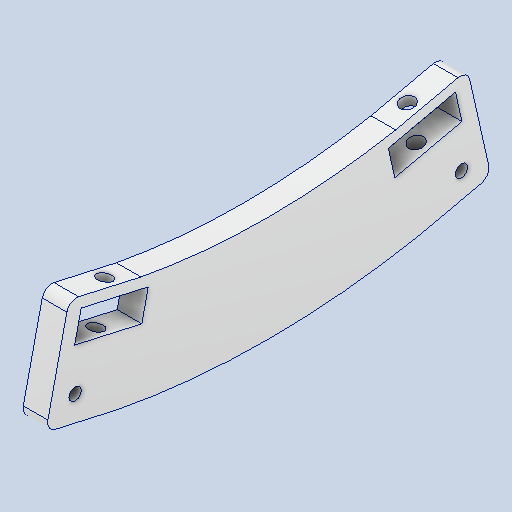
# Autodesk Inventor part: belt_liner_v2_Plate_14
Saved by Autodesk Inventor 2025.2 (Build 292293000, 293)
## iProperties
Created: 2025-01-06
Part Number: belt_liner_v2_Plate_14
Material: アルミニウム 6061
Document SubType Name: Modeling
Designer: haruy
Density: 2.7 g/cm^3
Appearance: アルミニウム - フラット
Mass: 22.219 g
Surface Area: 51.7738 cm^2
Volume: 8.22926 cm^3
Author: haruy
Autodesk Inventor part; units mm, degrees
ref_plane "YZ Plane" through (0, 0, 0) normal (1, 0, 0) x (0, 1, 0)
ref_plane "XZ Plane" through (0, 0, 0) normal (0, 1, 0) x (-1, 0, 0)
ref_plane "XY Plane" through (0, 0, 0) normal (0, 0, 1) x (1, 0, 0)
derived "base_weel-v2-Sketch-Base.ipt"
sketch "スケッチ1" plane through (0, 0, 0) normal (1, 0, 0) x (0, 1, 0)
  line L0 (-315, 315) -> (315, 315)
  line L1 (315, 315) -> (315, -315)
  line L2 (315, -315) -> (-315, -315)
  line L3 (-315, -315) -> (-315, 315)
  line L4 (-315, 315) -> (315, -315) construction
  line L5 (315, 315) -> (-315, -315) construction
  line L6 (-295, 218) -> (-295, -202)
  line L7 (-295, -202) -> (-315, -202)
  line L8 (-315, -202) -> (-315, 210)
  line L9 (242, 315) -> (-242, 315)
  line L10 (-242, 315) -> (-242, 295)
  line L11 (-242, 295) -> (242, 295)
  line L12 (242, 295) -> (242, 315)
  line L13 (-295, 218) -> (-295, 315)
  line L14 (0, 0) -> (-956.5973, 0)
  circle A0 centre (0, 0) radius 400
  line L15 (-330, 25) -> (-380, 25)
  line L16 (-380, 25) -> (-380, -25)
  line L17 (-380, -25) -> (-330, -25)
  line L18 (-330, -25) -> (-330, 25)
  line L19 (0, 0) -> (0, -630.9179)
  line L20 (-315, 40) -> (-395, 40)
  line L21 (-395, 40) -> (-395, 30)
  line L22 (-395, 30) -> (-315, 30)
  line L23 (-315, 30) -> (-315, 40)
  line L24 (-395, 30) -> (-385, 30)
  line L25 (-385, 30) -> (-385, 0)
  line L26 (-385, 0) -> (-395, 0)
  line L27 (-395, 0) -> (-395, 30)
  line L28 (295, 202) -> (315, 202)
  line L29 (315, 202) -> (315, -202)
  line L30 (315, -202) -> (295, -202)
  line L31 (295, -202) -> (295, 202)
  line L32 (-222.2183, -315) -> (242, -315)
  line L33 (242, -315) -> (242, -295)
  line L34 (242, -295) -> (-242, -295)
  line L35 (315, 315) -> (0, 0)
  line L36 (315, 125) -> (315, 145)
  circle A1 centre (512, 0) radius 122.5
  circle A2 centre (179.6905, 0) radius 600
  circle A3 centre (541.6815, 0) radius 200
  circle A4 centre (0, 0) radius 10
  arc A5 (0, 150) -> (0, -150) centre (0, 0) ccw
  arc A6 (0, 140) -> (0, -140) centre (0, 0) ccw
  line L37 (-146.3272, 32.9904) -> (-136.572, 30.791)
  line L38 (-137.5812, 37.6817) -> (-140.4404, 25)
  line L39 (-140.4404, 25) -> (-145.318, 26.0997)
  line L40 (-145.318, 26.0997) -> (-142.4588, 38.7814)
  line L41 (-142.4588, 38.7814) -> (-137.5812, 37.6817)
  arc A7 (-29.1302, 142.0438) -> (-29.1302, -142.0438) centre (0, 0) ccw
  circle A8 centre (-151.4904, 39.2799) radius 6.5 construction
  circle A9 centre (-129.0401, 34.2184) radius 6.5 construction
  circle A10 centre (-129.0401, 34.2184) radius 1.5 construction
  circle A11 centre (-151.4904, 39.2799) radius 1.5 construction
  line L42 (-30.1668, 22.5) -> (-174.1362, 22.5)
  line L43 (-174.1362, 22.5) -> (-174.1362, 7.5)
  line L44 (-174.1362, 7.5) -> (-30.1668, 7.5)
  line L45 (-30.1668, 7.5) -> (-30.1668, 22.5)
  circle A12 centre (-129.0401, -34.2184) radius 6.5 construction
  circle A13 centre (-129.0401, -34.2184) radius 1.5 construction
  line L46 (-142.4588, -38.7814) -> (-137.5812, -37.6817)
  line L47 (-145.318, -26.0997) -> (-142.4588, -38.7814)
  line L48 (-137.5812, -37.6817) -> (-140.4404, -25)
  line L49 (-140.4404, -25) -> (-145.318, -26.0997)
  circle A14 centre (-151.4904, -39.2799) radius 6.5 construction
  circle A15 centre (-151.4904, -39.2799) radius 1.5 construction
  line L50 (-146.3272, -32.9904) -> (-136.572, -30.791)
  line L51 (-30.1668, -22.5) -> (-174.1362, -22.5)
  line L52 (-174.1362, -7.5) -> (-30.1668, -7.5)
  line L53 (-30.1668, -7.5) -> (-30.1668, -22.5)
  line L54 (-174.1362, -22.5) -> (-174.1362, -7.5)
  line L55 (-151.4904, 39.2799) -> (-129.0401, 34.2184) construction
  line L56 (-129.0401, 34.2184) -> (-129.59, 31.7796) construction
  line L57 (-129.59, 31.7796) -> (-152.0402, 36.8412) construction
  line L58 (-152.0402, 36.8412) -> (-151.4904, 39.2799) construction
  line L59 (-129.0401, 34.2184) -> (-151.4904, 39.2799) construction
  line L60 (-151.4904, 39.2799) -> (-150.9405, 41.7187) construction
  line L61 (-150.9405, 41.7187) -> (-128.4903, 36.6572) construction
  line L62 (-128.4903, 36.6572) -> (-129.0401, 34.2184) construction
  line L63 (-128.4903, 36.6572) -> (-129.59, 31.7796) construction
  line L64 (-129.59, 31.7796) -> (-117.8838, 29.1404) construction
  line L65 (-117.8838, 29.1404) -> (-116.7841, 34.0179) construction
  line L66 (-116.7841, 34.0179) -> (-128.4903, 36.6572) construction
  line L67 (-150.9405, 41.7187) -> (-152.0402, 36.8412) construction
  line L68 (-152.0402, 36.8412) -> (-163.7464, 39.4804) construction
  line L69 (-163.7464, 39.4804) -> (-162.6467, 44.358) construction
  line L70 (-162.6467, 44.358) -> (-150.9405, 41.7187) construction
  line L71 (-155.2683, 45.2572) -> (-128.9412, 39.3216)
  line L72 (-128.9412, 39.3216) -> (-132.2403, 24.6889)
  line L73 (-132.2403, 24.6889) -> (-158.5673, 30.6245)
  line L74 (-158.5673, 30.6245) -> (-155.2683, 45.2572)
  line L75 (-128.9412, -39.3216) -> (-132.2403, -24.6889)
  line L76 (-155.2683, -45.2572) -> (-128.9412, -39.3216)
  line L77 (-132.2403, -24.6889) -> (-158.5673, -30.6245)
  line L78 (-158.5673, -30.6245) -> (-155.2683, -45.2572)
  arc A16 (-132.2403, 24.6889) -> (-132.2403, -24.6889) centre (0, 0) ccw
  arc A17 (-158.5673, 30.6245) -> (-158.5673, -30.6245) centre (0, 0) ccw
  circle A18 centre (-152.5, 15) radius 1.25
  line L79 (-145, 0) -> (-145, 74.7382) construction
  circle A19 centre (-137.5, 15) radius 1.25
  circle A20 centre (-137.5, -15) radius 1.25
  circle A21 centre (-152.5, -15) radius 1.25
  circle A22 centre (-151.4904, 39.2799) radius 1.25
  circle A23 centre (-129.0401, 34.2184) radius 1.25
  line L80 (-136.9835, 38.0595) -> (-140.0626, 24.4023)
  line L81 (-140.0626, 24.4023) -> (-145.9157, 25.7219)
  line L82 (-145.9157, 25.7219) -> (-142.8366, 39.3791)
  line L83 (-142.8366, 39.3791) -> (-136.9835, 38.0595)
  circle A24 centre (-151.4904, -39.2799) radius 1.25
  circle A25 centre (-129.0401, -34.2184) radius 1.25
  line L84 (-136.9835, -38.0595) -> (-140.0626, -24.4023)
  line L85 (-140.0626, -24.4023) -> (-145.9157, -25.7219)
  line L86 (-145.9157, -25.7219) -> (-142.8366, -39.3791)
  line L87 (-142.8366, -39.3791) -> (-136.9835, -38.0595)
  line L88 (0, 0) -> (0, 140)
  line L89 (0, 0) -> (-47.8828, 131.557)
  line L90 (0, 140) -> (0, 150)
  line L91 (-137.5846, 25.8938) -> (-134.2855, 40.5265)
  line L92 (-137.5846, -25.8938) -> (-134.2855, -40.5265)
  circle A26 centre (0, 0) radius 20
  line L93 (295, 45) -> (-295, 45)
  line L94 (-295, 45) -> (-295, 25)
  line L95 (-295, 25) -> (295, 25)
  line L96 (295, 25) -> (295, 45)
  line L97 (-40, 295) -> (-50, 295)
  line L98 (-50, 295) -> (-50, 45)
  line L99 (-50, 45) -> (-40, 45)
  line L100 (-40, 45) -> (-40, 295)
  line L101 (-50, -295) -> (-50, -45)
  line L102 (-40, -45) -> (-40, -295)
  line L103 (295, -45) -> (-295, -45)
  line L104 (-295, -25) -> (295, -25)
  line L105 (-40, 45) -> (-40, -45)
  line L106 (40, 45) -> (40, -45)
  circle A27 centre (20, 35) radius 1.5
  circle A28 centre (-20, 35) radius 1.5
  circle A29 centre (-20, -35) radius 1.5
  circle A30 centre (20, -35) radius 1.5
  circle A31 centre (-45, 125) radius 1.5
  circle A32 centre (-45, 125) radius 5
  circle A33 centre (-130, 35) radius 5
  circle A34 centre (-130, 35) radius 1.5
  line L107 (-40, 134.1641) -> (-40, 125)
  line L108 (-50, 125) -> (-50, 130.767)
  line L109 (-137.7498, 25) -> (-127.5801, 30.6246)
  line L110 (-132.5707, 45) -> (-126.366, 38.4342)
  line L111 (-40, -134.1641) -> (-40, -125)
  circle A35 centre (-45, -125) radius 5
  circle A36 centre (-45, -125) radius 1.5
  line L112 (-50, -125) -> (-50, -130.767)
  line L113 (-132.5707, -45) -> (-126.366, -38.4342)
  circle A37 centre (-130, -35) radius 5
  circle A38 centre (-130, -35) radius 1.5
  line L114 (-137.7498, -25) -> (-127.5801, -30.6246)
  line L115 (-242, -295) -> (-242, -315)
  line L116 (242, 315) -> (222, 315)
  line L117 (222, 315) -> (222, 295)
  line L118 (222, 295) -> (242, 295)
  line L119 (242, 295) -> (242, 315)
  line L120 (242, -315) -> (222, -315)
  line L121 (222, -315) -> (222, -295)
  line L122 (222, -295) -> (242, -295)
  line L123 (242, -295) -> (242, -315)
  line L124 (197, 295) -> (295, 197)
  line L125 (295, 197) -> (284.3934, 186.3934)
  line L126 (284.3934, 186.3934) -> (186.3934, 284.3934)
  line L127 (186.3934, 284.3934) -> (197, 295)
  line L128 (197, 295) -> (197, 315)
  line L129 (197.9167, 294.0833) -> (187.3101, 283.4767)
  line L130 (198.2703, 272.5165) -> (272.5165, 198.2703)
  line L131 (272.5165, 198.2703) -> (231.5043, 157.2581)
  line L132 (231.5043, 157.2581) -> (157.2581, 231.5043)
  line L133 (157.2581, 231.5043) -> (198.2703, 272.5165)
  line L134 (290.9013, 201.0987) -> (280.2947, 190.4921)
  line L135 (93.7624, 295) -> (295, 93.7624)
  line L136 (295, 93.7624) -> (284.3934, 83.1558)
  line L137 (284.3934, 83.1558) -> (83.1558, 284.3934)
  line L138 (214.1802, 277.8198) -> (203.5736, 267.2132)
  line L139 (277.8198, 214.1802) -> (267.2132, 203.5736)
  circle A39 centre (199.6845, 281.7089) radius 1.5
  circle A40 centre (213.8266, 267.5668) radius 1.5
  line L140 (186.3934, 284.3934) -> (175.7868, 295)
  circle A41 centre (187, 305) radius 1.5
  circle A42 centre (177, 305) radius 1.5
  line L141 (172, 315) -> (172, 295)
  line L142 (93.7624, 295) -> (93.7624, 295)
  line L143 (93.7624, 295) -> (93.7624, 315)
  line L144 (83.1558, 284.3934) -> (72.5492, 295)
  line L145 (68.7624, 315) -> (68.7624, 295)
  line L146 (284.3934, 186.3934) -> (295, 175.7868)
  line L147 (295, 197) -> (315, 197)
  line L148 (295, 93.7624) -> (295, 93.7624)
  line L149 (284.3934, 83.1558) -> (295, 72.5492)
  line L150 (-197, 295) -> (-197, 315)
  line L151 (-172, 315) -> (-172, 295)
  line L152 (-93.7624, 295) -> (-93.7624, 315)
  line L153 (-68.7624, 315) -> (-68.7624, 295)
  line L154 (-83.1558, 284.3934) -> (-72.5492, 295)
  line L155 (-93.7624, 295) -> (-295, 93.7624)
  line L156 (-83.1558, 284.3934) -> (-93.7624, 295)
  line L157 (-284.3934, 83.1558) -> (-83.1558, 284.3934)
  line L158 (-295, 93.7624) -> (-284.3934, 83.1558)
  line L159 (-284.3934, 83.1558) -> (-295, 72.5492)
  line L160 (-272.5165, 198.2703) -> (-231.5043, 157.2581)
  line L161 (-157.2581, 231.5043) -> (-198.2703, 272.5165)
  line L162 (-284.3934, 186.3934) -> (-186.3934, 284.3934)
  line L163 (-186.3934, 284.3934) -> (-175.7868, 295)
  line L164 (-197, 295) -> (-295, 197)
  line L165 (-197.9167, 294.0833) -> (-187.3101, 283.4767)
  line L166 (-214.1802, 277.8198) -> (-203.5736, 267.2132)
  line L167 (-290.9013, 201.0987) -> (-280.2947, 190.4921)
  line L168 (-284.3934, 186.3934) -> (-295, 175.7868)
  line L169 (-295, 197) -> (-315, 197)
  line L170 (-93.7624, -295) -> (-295, -93.7624)
  line L171 (-284.3934, -83.1558) -> (-83.1558, -284.3934)
  line L172 (-295, -93.7624) -> (-284.3934, -83.1558)
  line L173 (-197, -295) -> (-295, -197)
  line L174 (-284.3934, -186.3934) -> (-186.3934, -284.3934)
  line L175 (-290.9013, -201.0987) -> (-280.2947, -190.4921)
  line L176 (-214.1802, -277.8198) -> (-203.5736, -267.2132)
  line L177 (-197.9167, -294.0833) -> (-187.3101, -283.4767)
  line L178 (-83.1558, -284.3934) -> (-93.7624, -295)
  line L179 (284.3934, -83.1558) -> (83.1558, -284.3934)
  line L180 (83.1558, -284.3934) -> (93.7624, -295)
  line L181 (93.7624, -295) -> (295, -93.7624)
  line L182 (284.3934, -186.3934) -> (186.3934, -284.3934)
  line L183 (197.9167, -294.0833) -> (187.3101, -283.4767)
  line L184 (197, -295) -> (295, -197)
  line L185 (290.9013, -201.0987) -> (280.2947, -190.4921)
  line L186 (295, -93.7624) -> (284.3934, -83.1558)
  line L187 (242, 295) -> (222, 295)
  arc A43 (0, 86) -> (0, -86) centre (0, 0) ccw
  circle A44 centre (-90.8667, 48.5) radius 21
  circle A45 centre (0, 0) radius 124
  circle A46 centre (-90.8667, 48.5) radius 17
  arc A47 (40.4951, 75.8693) -> (0, 86) centre (0, 0) ccw
  line L188 (-40, 45) -> (-50, 45)
  line L189 (-50, 45) -> (-50, -45)
  line L190 (-50, -45) -> (-40, -45)
  line L191 (-40, -45) -> (-40, 45)
  line L192 (-40, 295) -> (-50, 295)
  line L193 (-50, 295) -> (-50, 315)
  line L194 (-50, 315) -> (-40, 315)
  line L195 (-40, 315) -> (-40, 295)
  line L196 (-40, -295) -> (-50, -295)
  line L197 (-50, -295) -> (-50, -315)
  line L198 (-50, -315) -> (-40, -315)
  line L199 (-40, -315) -> (-40, -295)
  line L200 (40, -315) -> (40, -295)
  line L201 (50, -295) -> (50, -315)
  line L202 (50, -295) -> (50, -45)
  line L203 (40, -45) -> (40, -295)
  line L204 (40, -45) -> (40, 45)
  line L205 (50, 45) -> (50, -45)
  line L206 (40, 45) -> (40, 295)
  line L207 (50, 295) -> (50, 45)
  line L208 (40, 315) -> (40, 295)
  line L209 (50, 295) -> (50, 315)
  line L210 (-40.4092, 123.019) -> (-35, 135.5544)
  line L211 (-48.7417, 121.6834) -> (-55, 128.7439)
  line L212 (-40.4092, -123.019) -> (-35, -135.5544)
  line L213 (-48.7417, -121.6834) -> (-55, -128.7439)
  arc A48 (40.4951, 75.8693) -> (-40.4951, -75.8693) centre (0, 0) ccw
  circle A49 centre (0, 0) radius 86 construction
  circle A50 centre (0, 0) radius 78.5
  circle A51 centre (-45, 58) radius 1.5
  circle A52 centre (-45, 58) radius 5
  circle A53 centre (45, 58) radius 5
  circle A54 centre (45, 58) radius 1.5
  line L214 (46.5549, 53.2479) -> (55, 56.0112)
  line L215 (40.325, 56.2267) -> (35, 70.2656)
  line L216 (50, 60.5165) -> (50, 69.9714)
  arc A55 (50, 69.9714) -> (40.4951, 75.8693) centre (0, 0) ccw
  line L217 (-40.325, 56.2267) -> (-35, 70.2656)
  line L218 (-46.5549, 53.2479) -> (-55, 56.0112)
  line L219 (-40.325, -56.2267) -> (-35, -70.2656) construction
  circle A56 centre (-45, -58) radius 5
  line L220 (-46.5549, -53.2479) -> (-55, -56.0112)
  circle A57 centre (-45, -58) radius 1.5
  line L221 (-40, -67.5444) -> (-40, -76.1315)
  arc A58 (-40.526, -75.8528) -> (-40, -76.1315) centre (0, 0) ccw
  line L222 (-40, -76.1315) -> (-40, -58)
  line L223 (222.6655, 269.3345) -> (212.0589, 258.7279)
  line L224 (269.3345, 222.6655) -> (258.7279, 212.0589)
  circle A59 centre (267.5668, 213.8266) radius 1.5
  circle A60 centre (281.7089, 199.6845) radius 1.5
  line L225 (294.0833, 197.9167) -> (283.4767, 187.3101)
  line L226 (315, 172) -> (295, 172)
  circle A61 centre (305, 177) radius 1.5
  circle A62 centre (305, 187) radius 1.5
  line L227 (295, 197) -> (315, 197)
  circle A63 centre (83.7624, 305) radius 1.5
  circle A64 centre (73.7624, 305) radius 1.5
  line L228 (197.9167, 294.0833) -> (94.6791, 294.0833)
  line L229 (187.3101, 283.4767) -> (84.0725, 283.4767)
  line L230 (94.6791, 294.0833) -> (84.0725, 283.4767)
  circle A65 centre (96.4469, 281.7089) radius 1.5
  circle A66 centre (110.5891, 267.5668) radius 1.5
  line L231 (119.4279, 269.3345) -> (108.8213, 258.7279)
  line L232 (295, 93.7624) -> (315, 93.7624)
  line L233 (315, 68.7624) -> (295, 68.7624)
  circle A67 centre (305, 73.7624) radius 1.5
  circle A68 centre (305, 83.7624) radius 1.5
  line L234 (294.0833, 94.6791) -> (283.4767, 84.0725)
  circle A69 centre (281.7089, 96.4469) radius 1.5
  circle A70 centre (267.5668, 110.5891) radius 1.5
  line L235 (269.3345, 119.4279) -> (258.7279, 108.8213)
  line L236 (-197, 295) -> (-197, 315)
  line L237 (-172, 315) -> (-172, 295)
  circle A71 centre (-177, 305) radius 1.5
  circle A72 centre (-187, 305) radius 1.5
  line L238 (-197.9167, 294.0833) -> (-187.3101, 283.4767)
  circle A73 centre (-199.6845, 281.7089) radius 1.5
  line L239 (-214.1802, 277.8198) -> (-203.5736, 267.2132)
  circle A74 centre (-213.8266, 267.5668) radius 1.5
  line L240 (-222.6655, 269.3345) -> (-212.0589, 258.7279)
  circle A75 centre (-267.5668, 213.8266) radius 1.5
  line L241 (-269.3345, 222.6655) -> (-258.7279, 212.0589)
  circle A76 centre (-281.7089, 199.6845) radius 1.5
  line L242 (-294.0833, 197.9167) -> (-283.4767, 187.3101)
  line L243 (-295, 197) -> (-315, 197)
  circle A77 centre (-305, 187) radius 1.5
  circle A78 centre (-305, 177) radius 1.5
  line L244 (-315, 172) -> (-295, 172)
  line L245 (-295, 93.7624) -> (-315, 93.7624)
  line L246 (-315, 68.7624) -> (-295, 68.7624)
  circle A79 centre (-305, 73.7624) radius 1.5
  circle A80 centre (-305, 83.7624) radius 1.5
  line L247 (-294.0833, 94.6791) -> (-283.4767, 84.0725)
  circle A81 centre (-281.7089, 96.4469) radius 1.5
  circle A82 centre (-267.5668, 110.5891) radius 1.5
  line L248 (-269.3345, 119.4279) -> (-258.7279, 108.8213)
  line L249 (-119.4279, 269.3345) -> (-108.8213, 258.7279)
  circle A83 centre (-110.5891, 267.5668) radius 1.5
  circle A84 centre (-96.4469, 281.7089) radius 1.5
  line L250 (-94.6791, 294.0833) -> (-84.0725, 283.4767)
  line L251 (-93.7624, 295) -> (-93.7624, 315)
  line L252 (-68.7624, 315) -> (-68.7624, 295)
  circle A85 centre (-73.7624, 305) radius 1.5
  circle A86 centre (-83.7624, 305) radius 1.5
  line L253 (-295, -197) -> (-315, -197)
  circle A87 centre (-305, -187) radius 1.5
  circle A88 centre (-305, -177) radius 1.5
  line L254 (-315, -172) -> (-295, -172)
  line L255 (-294.0833, -197.9167) -> (-283.4767, -187.3101)
  circle A89 centre (-281.7089, -199.6845) radius 1.5
  circle A90 centre (-267.5668, -213.8266) radius 1.5
  line L256 (-269.3345, -222.6655) -> (-258.7279, -212.0589)
  line L257 (-222.6655, -269.3345) -> (-212.0589, -258.7279)
  circle A91 centre (-213.8266, -267.5668) radius 1.5
  circle A92 centre (-199.6845, -281.7089) radius 1.5
  line L258 (-197.9167, -294.0833) -> (-187.3101, -283.4767)
  line L259 (-197, -295) -> (-197, -315)
  circle A93 centre (-187, -305) radius 1.5
  circle A94 centre (-177, -305) radius 1.5
  line L260 (-172, -315) -> (-172, -295)
  line L261 (-295, -93.7624) -> (-315, -93.7624)
  circle A95 centre (-305, -83.7624) radius 1.5
  circle A96 centre (-305, -73.7624) radius 1.5
  line L262 (-315, -68.7624) -> (-295, -68.7624)
  line L263 (-294.0833, -94.6791) -> (-283.4767, -84.0725)
  circle A97 centre (-281.7089, -96.4469) radius 1.5
  circle A98 centre (-267.5668, -110.5891) radius 1.5
  line L264 (-269.3345, -119.4279) -> (-258.7279, -108.8213)
  line L265 (-119.4279, -269.3345) -> (-108.8213, -258.7279)
  circle A99 centre (-110.5891, -267.5668) radius 1.5
  circle A100 centre (-96.4469, -281.7089) radius 1.5
  line L266 (-94.6791, -294.0833) -> (-84.0725, -283.4767)
  line L267 (-93.7624, -295) -> (-93.7624, -315)
  circle A101 centre (-83.7624, -305) radius 1.5
  circle A102 centre (-73.7624, -305) radius 1.5
  line L268 (-68.7624, -315) -> (-68.7624, -295)
  line L269 (68.7624, -315) -> (68.7624, -295)
  circle A103 centre (73.7624, -305) radius 1.5
  circle A104 centre (83.7624, -305) radius 1.5
  line L270 (93.7624, -295) -> (93.7624, -315)
  line L271 (94.6791, -294.0833) -> (84.0725, -283.4767)
  circle A105 centre (96.4469, -281.7089) radius 1.5
  circle A106 centre (110.5891, -267.5668) radius 1.5
  line L272 (119.4279, -269.3345) -> (108.8213, -258.7279)
  line L273 (172, -315) -> (172, -295)
  circle A107 centre (177, -305) radius 1.5
  circle A108 centre (187, -305) radius 1.5
  line L274 (197, -295) -> (197, -315)
  line L275 (197.9167, -294.0833) -> (187.3101, -283.4767)
  circle A109 centre (199.6845, -281.7089) radius 1.5
  circle A110 centre (213.8266, -267.5668) radius 1.5
  line L276 (222.6655, -269.3345) -> (212.0589, -258.7279)
  line L277 (269.3345, -222.6655) -> (258.7279, -212.0589)
  circle A111 centre (267.5668, -213.8266) radius 1.5
  circle A112 centre (281.7089, -199.6845) radius 1.5
  line L278 (294.0833, -197.9167) -> (283.4767, -187.3101)
  line L279 (295, -197) -> (315, -197)
  circle A113 centre (305, -187) radius 1.5
  circle A114 centre (305, -177) radius 1.5
  line L280 (315, -172) -> (295, -172)
  line L281 (295, -93.7624) -> (315, -93.7624)
  circle A115 centre (305, -83.7624) radius 1.5
  circle A116 centre (305, -73.7624) radius 1.5
  line L282 (315, -68.7624) -> (295, -68.7624)
  line L283 (294.0833, -94.6791) -> (283.4767, -84.0725)
  circle A117 centre (281.7089, -96.4469) radius 1.5
  line L284 (269.3345, -119.4279) -> (258.7279, -108.8213)
  circle A118 centre (267.5668, -110.5891) radius 1.5
  line L285 (-295, 202) -> (-315, 202)
  line L286 (265, 45) -> (265, 25)
  circle A119 centre (275, 35) radius 1.5
  circle A120 centre (285, 35) radius 1.5
  circle A121 centre (305, 35) radius 1.5
  circle A122 centre (305, 25) radius 1.5
  line L287 (295, 25) -> (315, 25)
  line L288 (265, -45) -> (265, -25)
  circle A123 centre (275, -35) radius 1.5
  circle A124 centre (285, -35) radius 1.5
  circle A125 centre (305, -35) radius 1.5
  circle A126 centre (305, -25) radius 1.5
  circle A127 centre (-305, -25) radius 1.5
  circle A128 centre (-305, -35) radius 1.5
  circle A129 centre (-285, -35) radius 1.5
  circle A130 centre (-275, -35) radius 1.5
  line L289 (-265, -45) -> (-265, -25)
  line L290 (-265, 45) -> (-265, 25)
  circle A131 centre (-275, 35) radius 1.5
  circle A132 centre (-285, 35) radius 1.5
  circle A133 centre (-305, 35) radius 1.5
  circle A134 centre (-305, 25) radius 1.5
  circle A135 centre (48, 345) radius 44
  circle A136 centre (-50, 345) radius 44
  circle A137 centre (-50, 345) radius 15
  line L291 (295, 45) -> (315, 45)
  line L292 (295, 15) -> (315, 15)
  line L293 (-315, 45.5) -> (-390, 45.5)
  line L294 (-390, 45.5) -> (-390, 0)
  line L295 (-390, 0) -> (-315, 0)
  line L296 (-315, 0) -> (-315, 45.5)
  circle A138 centre (-305, 48) radius 1.5
  circle A139 centre (-305, -48) radius 1.5
  line L297 (114.7878, 210) -> (54.7878, 210)
  line L298 (54.7878, 210) -> (54.7878, 270)
  line L299 (54.7878, 270) -> (114.7878, 270)
  line L300 (114.7878, 270) -> (114.7878, 210)
  line L301 (34.7878, 210) -> (-25.2122, 210)
  line L302 (-25.2122, 210) -> (-25.2122, 270)
  line L303 (-25.2122, 270) -> (34.7878, 270)
  line L304 (34.7878, 270) -> (34.7878, 210)
  line L305 (-45.2122, 250) -> (-115.2122, 250)
  line L306 (-115.2122, 250) -> (-115.2122, 266)
  line L307 (-115.2122, 266) -> (-45.2122, 266)
  line L308 (-45.2122, 266) -> (-45.2122, 250)
  line L309 (-50.2122, 214) -> (-110.2122, 214)
  line L310 (-110.2122, 214) -> (-110.2122, 230)
  line L311 (-110.2122, 230) -> (-50.2122, 230)
  line L312 (-50.2122, 230) -> (-50.2122, 214)
  circle A140 centre (0, 0) radius 175.5
  line L313 (-185, -89) -> (-302, -89)
  line L314 (-302, -89) -> (-302, 89)
  line L315 (-302, 89) -> (-185, 89)
  line L316 (-185, 89) -> (-185, -89)
  line L317 (287, -17.7878) -> (205, -17.7878)
  line L318 (205, -17.7878) -> (205, 79.2122)
  line L319 (205, 79.2122) -> (287, 79.2122)
  line L320 (287, 79.2122) -> (287, -17.7878)
  line L321 (284.5, -114.7878) -> (207.5, -114.7878)
  line L322 (207.5, -114.7878) -> (207.5, -37.7878)
  line L323 (207.5, -37.7878) -> (284.5, -37.7878)
  line L324 (284.5, -37.7878) -> (284.5, -114.7878)
  line L325 (281, 99.2122) -> (211, 99.2122)
  line L326 (211, 99.2122) -> (211, 115.2122)
  line L327 (211, 115.2122) -> (281, 115.2122)
  line L328 (281, 115.2122) -> (281, 99.2122)
  line L329 (137.7122, 315) -> (-137.7122, 315)
  line L330 (-137.7122, 315) -> (-137.7122, 185)
  line L331 (-137.7122, 185) -> (137.7122, 185)
  line L332 (137.7122, 185) -> (137.7122, 315)
  line L333 (315, -137.7122) -> (185, -137.7122)
  line L334 (185, -137.7122) -> (185, 137.7122)
  line L335 (185, 137.7122) -> (315, 137.7122)
  line L336 (315, 137.7122) -> (315, -137.7122)
  line L337 (258.7782, 137.7122) -> (278.7782, 137.7122)
  line L338 (278.7782, 137.7122) -> (278.7782, 127.7122)
  line L339 (278.7782, 127.7122) -> (258.7782, 127.7122)
  line L340 (258.7782, 127.7122) -> (258.7782, 137.7122)
  circle A141 centre (268.7782, 132.7122) radius 1.5
  line L341 (278.7782, 137.7122) -> (231.1981, 137.7122)
  line L342 (231.1981, 137.7122) -> (231.1981, 147.7122)
  line L343 (231.1981, 147.7122) -> (278.7782, 147.7122)
  line L344 (278.7782, 147.7122) -> (278.7782, 137.7122)
  line L345 (255.1924, 112.3568) -> (233.9792, 133.57)
  line L346 (233.9792, 133.57) -> (230.4437, 130.0345)
  line L347 (230.4437, 130.0345) -> (251.6569, 108.8213)
  line L348 (251.6569, 108.8213) -> (255.1924, 112.3568)
  line L349 (288.78, 89.3758) -> (114.1246, 264.0312)
  line L350 (269.3345, 126.499) -> (265.799, 122.9634)
  line L351 (248.1213, 147.7122) -> (269.3345, 126.499)
  line L352 (244.5858, 144.1766) -> (248.1213, 147.7122)
  circle A142 centre (268.7782, 132.7122) radius 4
  line L353 (233.9792, 133.57) -> (244.5858, 144.1766)
  line L354 (-330, 143.5) -> (-340, 143.5)
  line L355 (-340, 143.5) -> (-340, -143.5)
  line L356 (-340, -143.5) -> (-330, -143.5)
  line L357 (-330, -143.5) -> (-330, 143.5)
  line L358 (-315, 119) -> (-295, 119)
  line L359 (-295, 119) -> (-295, 104)
  line L360 (-295, 104) -> (-315, 104)
  line L361 (-315, 104) -> (-315, 119)
  line L362 (-315, 153.5) -> (-325, 153.5)
  line L363 (-325, 153.5) -> (-325, 0)
  line L364 (-325, 0) -> (-315, 0)
  line L365 (-315, 0) -> (-315, 153.5)
  line L366 (-340, 133.5) -> (-345, 133.5)
  line L367 (-345, 133.5) -> (-345, 143.5)
  line L368 (-345, 143.5) -> (-340, 143.5)
  line L369 (-340, 143.5) -> (-340, 133.5)
  line L370 (-330, 133.5) -> (-325, 133.5)
  line L371 (-325, 133.5) -> (-325, 143.5)
  line L372 (-325, 143.5) -> (-330, 143.5)
  line L373 (-330, 143.5) -> (-330, 133.5)
  line L374 (-325, 153.5) -> (-345, 153.5)
  line L375 (-345, 153.5) -> (-345, 143.5)
  line L376 (-345, 143.5) -> (-325, 143.5)
  line L377 (-325, 143.5) -> (-325, 153.5)
  line L378 (-295, 104) -> (-345, 104)
  line L379 (-345, 104) -> (-345, 98)
  line L380 (-345, 98) -> (-295, 98)
  line L381 (-295, 98) -> (-295, 104)
  line L382 (185, -25) -> (180, -25)
  line L383 (180, -25) -> (180, -15)
  line L384 (180, -15) -> (185, -15)
  line L385 (185, -15) -> (185, -25)
  line L386 (185, -25) -> (195, -25)
  line L387 (195, -25) -> (195, -15)
  line L388 (195, -15) -> (185, -15)
  line L389 (185, -15) -> (185, -25)
  line L390 (40, 180) -> (30, 180)
  line L391 (30, 180) -> (30, 195)
  line L392 (30, 195) -> (40, 195)
  line L393 (40, 195) -> (40, 180)
  circle A143 centre (-132.7122, 268.7782) radius 1.5
  circle A144 centre (132.7122, 268.7782) radius 1.5
  line L394 (-243.5, 89) -> (-243.5, -89)
  circle A145 centre (-214, 35) radius 1.5
  circle A146 centre (-214, -35) radius 1.5
  line L395 (-214, 89) -> (-214, -89)
  line L396 (-246, 89) -> (-246, -89)
  circle A147 centre (-254.5, 35) radius 4
  circle A148 centre (-254.5, -35) radius 4
  circle A149 centre (0, 0) radius 100
  circle A150 centre (-134.1671, -14.9726) radius 5
  circle A151 centre (-134.1671, -14.9726) radius 1.25
  circle A152 centre (-134.9074, -5) radius 5
  circle A153 centre (-134.9074, -5) radius 1.25
  point P0 (-141.4496, 31.8907)
  point P1 (-137.5846, 25.8938)
  point P2 (-137.5846, -25.8938)
  point P3 (-129.8839, -35.1407)
  point P4 (-130.198, -33.7474)
  point P5 (-130.198, 33.7474)
  point P6 (-129.8839, 35.1407)
  point P7 (-150, 0)
  point P8 (-242, 305)
  point P9 (-295, 93.7624)
  point P10 (-161.4975, 0)
  point P11 (305, 25)
  point P12 (295, 35)
  dimension "d1" = 2.5
  dimension "d2" = 2.5
  dimension "d3" = 0.5
  measures "d1" diameter of A22
  measures "d2" diameter of A23
  measures "d3" distance between parallel lines of L41 L83
ref_plane "作業平面1" through (0, 0, 0) normal (1, 0, 0) x (0, 1, 0)
extrude "押し出し1" add sketch "スケッチ1" against normal blind 5 contours L103 L76 L78 | L78 L77 A5 L76 L103 | A5 L50 L86 L87 A7 L76 | A17 L104 A5 L77 | A17 L51 A5 L104 | L93 L71 A5 L73 L74 | L74 L71 L93 | A5 L77 L86 L50 | A7 L87 L84 L50 A6 L92 L76 | A5 L104 A7 L85 L86 L77 | A17 L52 A5 L51 | A5 L51 A7 L104 | L71 A7 L83 L82 L37 A5 | L73 A5 L95 A17 | L95 A5 L42 A17 | L92 A6 L76 | A6 L92 L77 L114 L75 A37 L76 | A5 L52 A7 L51 | A17 L14 A5 L52 | L104 L85 A7 | A7 L51 A6 L104 L84 L85 | L37 L82 L73 A5 | L71 L91 A6 L37 L80 L83 A7 | L73 L82 L81 A7 L95 A5 | L42 A5 L44 A17 | L95 A7 L42 A5 | L104 L77 L75 | L75 L114 L77 L104 | A6 L92 | A37 L75 A38 L76 | A17 L44 A5 L14 | A5 L14 A7 L52 | A7 L52 A6 L51 | L71 A6 L91 | L71 A33 L72 L109 L73 L91 A6 | L42 A7 L44 A5 | L95 L81 L80 A6 L42 A7 | A7 L81 L95 | L77 L104 A6 L51 A16 | L77 L114 L104 | L51 A6 A150 A16 | L84 L77 A6 L50 | L77 L84 L104 A6 | A6 L114 L77 | A5 L44 A7 L14 | A7 L14 A6 L52 | L91 A6 | L71 L72 A34 A33 | L42 A6 L44 A7 | A150 A16 A151 | A38 L75 A25 | A7 L44 A6 L14 | L52 A152 A150 A6 | A6 A152 L52 | L37 A6 L73 L80 | L73 L109 A6 | A6 L95 L80 L73 | L95 L73 L109 L72 | L72 L73 L95 | L42 A16 L44 A6 | A6 L95 L73 A16 L42 | A151 A16 | A16 A152 L52 | L52 A152 A16 A153 | A16 A150 A152 | A16 A152 L14 | L14 A6 L44 A16 | L14 A152 A6 | L109 L73 L95 | L72 A23 A34 | A153 A16 | A18 | A19 | A20 | A21 picked at (-136.0717, -12.8293) picked at (-130.8632, -35.5062) picked at (-134.2663, -14.9837) picked at (-137.3756, -7.8001) picked at (-136.3719, -7.0216) picked at (-130.8632, 35.5062) picked at (-135.0071, -5.0037)
sketch "スケッチ2" plane through (-5, -155.2683, 45.2572) normal (0, -0.9755144, 0.2199357) x (1, 0, 0)
  line L0 (5, 0) -> (0, 0) projected
  line L1 (5, 24.8819) -> (5, -108.7598) projected
  point P0 (5, -10)
  point P1 (2.5, -10)
  dimension "d6" = 10
  dimension "d7" = 2.5
  measures "d6" distance from line of L0 point (2.5, -10)
  measures "d7" distance from line of point (2.5, -10) L1
hole "穴1" at (-2.5, -157.4676, 35.5021) direction (0, 0.9755144, -0.2199357) diameter 3 end through all
sketch "スケッチ3" plane through (-5, -158.5673, -30.6245) normal (0, -0.9755144, -0.2199357) x (1, 0, 0)
  line L0 (5, -15) -> (0, -15) projected
  line L1 (5, 93.7598) -> (5, -39.8819) projected
  point P0 (5, -5)
  point P1 (2.5, -5)
  dimension "d15" = 10
  dimension "d16" = 2.5
  measures "d15" distance from line of point (2.5, -5) L0
  measures "d16" distance from line of point (2.5, -5) L1
hole "穴2" at (-2.5, -157.4676, -35.5021) direction (0, 0.9755144, 0.2199357) diameter 3 end through all
extrude "押し出し2" cut sketch "スケッチ1" against normal blind 5 contours L92 A6 L76 | A6 L92 L77 L114 L75 A37 L76 | L104 L77 L75 | L75 L114 L77 L104 | A37 L75 A38 L76 | L71 A6 L91 | L71 A33 L72 L109 L73 L91 A6 | L77 L104 A6 L51 A16 | L77 L114 L104 | L51 A6 A150 A16 | A6 L114 L77 | L71 L72 A34 A33 | A150 A16 A151 | A38 L75 A25 | L52 A152 A150 A6 | A6 A152 L52 | L73 L109 A6 | L95 L73 L109 L72 | L72 L73 L95 | L42 A16 L44 A6 | A6 L95 L73 A16 L42 | A151 A16 | A16 A152 L52 | L52 A152 A16 A153 | A16 A150 A152 | A16 A152 L14 | L14 A6 L44 A16 | L14 A152 A6 | L109 L73 L95 | L72 A23 A34 | A153 A16 | A19 | A20 picked at (-136.0717, -12.8293) picked at (-130.8632, -35.5062) picked at (-134.2663, -14.9837) picked at (-137.3756, -7.8001) picked at (-136.3719, -7.0216) picked at (-130.8632, 35.5062) picked at (-135.0071, -5.0037)
fillet "フィレット1" radius 2 4 edges at (-2.5, -155.2683, 45.2572) (-2.5, -134.2855, 40.5265) (-2.5, -134.2855, -40.5265) (-2.5, -155.2683, -45.2572)
